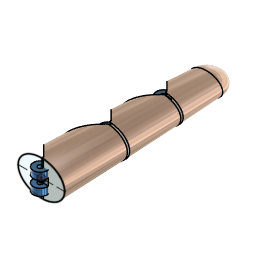
index finger assembly v3 (Autodesk Fusion 360 design; units mm, degrees)
Autodesk Fusion 360 part; units mm, degrees
sketch "base" plane through (0, 0, 0) normal (0, 1, 0) x (1, 0, 0) in component "index and ring finger part 2 v4"
  ellipse E0 centre (0, 0) end of major axis (9, 0) minor radius 6.5
  line L0 (-9, 0) -> (9, 0) construction
  line L1 (0, -6.5) -> (0, 6.5) construction
  dimension "d1" = 18
  dimension "d2" = 13
  constraint coincident E0 L0.start
  constraint coincident E0 L0.end
  constraint coincident E0 L1.start
  constraint coincident E0 L1.end
  constraint coincident E0.centre origin
  constraint horizontal L0
  measures "d1" distance of E0
ref_plane "WorkPlane1" through (0, 23, 0) normal (0, 1, 0) x (1, 0, 0) in component "index and ring finger part 2 v4"
sketch "top" plane through (0, 23, 0) normal (0, 1, 0) x (1, 0, 0) in component "index and ring finger part 2 v4"
  ellipse E0 centre (0, 0) end of major axis (8, 0) minor radius 5.5
  line L0 (-8, 0) -> (8, 0) construction
  line L1 (0, -5.5) -> (0, 5.5) construction
  dimension "d4" = 16
  dimension "d5" = 11
  constraint coincident E0 L0.start
  constraint coincident E0 L0.end
  constraint coincident E0 L1.start
  constraint coincident E0 L1.end
  constraint coincident E0.centre origin
  constraint horizontal L0
  measures "d4" distance of E0
loft "Loft1" add profiles "top", "base" section 1 section 2 makes body 1 in component "index and ring finger part 2 v4"
sketch "cut" plane through (0, 0, 0) normal (0, 0, 1) x (1, 0, 0) in component "index and ring finger part 2 v4"
  line L0 (0, 23) -> (0, 23.5)
  line L1 (0, 0) -> (0, 1)
  line L2 (0, 1) -> (-14.1421, 15.1421)
  line L3 (0, 1) -> (20, 1) construction
  line L4 (-14.1421, 15.1421) -> (-14.1421, 0)
  line L5 (-14.1421, 0) -> (0, 0)
  line L6 (0, 0) -> (0, -0.5)
  line L7 (0, 23) -> (0, 22)
  line L8 (0, 22) -> (-14.1421, 7.8579)
  line L9 (0, 22) -> (20, 22) construction
  line L10 (0, 23) -> (-11.4565, 23)
  line L11 (-11.4565, 23) -> (-14.1421, 7.8579)
  dimension "d6" = 0.5
  dimension "d7" = 1
  dimension "d8" = 135
  dimension "d9" = 20
  dimension "d10" = 0.5
  dimension "d11" = 1
  dimension "d12" = 135
  dimension "d13" = 20
  constraint vertical L0
  constraint coincident L1.start L5.end
  constraint vertical L1
  constraint horizontal L3
  constraint parallel L1 L4
  constraint perpendicular L1 L5
  constraint perpendicular L5 L6
  constraint parallel L0 L7
  constraint horizontal L9
  constraint perpendicular L7 L10
  measures "d6" distance of L0.start L0.end
  measures "d7" distance of L1.start L1.end
  measures "d8" angle of L2 L3
  measures "d9" distance of L1.end L2.end
  measures "d10" distance of L1.start L6.end
  measures "d11" distance of L0.start L7.end
  measures "d12" angle of L8 L9
  measures "d13" distance of L7.end L8.end
extrude "Extrude1" cut sketch "cut" along normal mid plane 40 contours L1 L2 L4 L5 L8 | L2 L7 L8 L10 L11 bodies 1 in component "index and ring finger part 2 v4"
sketch "wheel" plane through (0, 0, 0) normal (0, 0, 1) x (1, 0, 0) in component "index and ring finger part 2 v4"
  line L0 (0, 0) -> (0, -0.5)
  circle A0 centre (0, -0.5) radius 3
  circle A1 centre (0.0423, 23.5794) radius 3
  dimension "d16" = 0.5
  dimension "d17" = 6
  dimension "d18" = 6
  constraint coincident L0.start origin
  constraint vertical L0
  constraint coincident L0.end A0.centre
  measures "d16" distance of L0.start L0.end
  measures "d17" diameter of A0
  measures "d18" diameter of A1
extrude "Extrude2" add sketch "wheel" along normal mid plane 3 separate body contours A1 makes body 2 in component "index and ring finger part 2 v4"
extrude "Extrude3" cut sketch "wheel" along normal mid plane 3 contours A0 bodies 1 in component "index and ring finger part 2 v4"
sketch "lower wheel offset" plane through (0, 0, -1.5) normal (0, 0, 1) x (-1, 0, 0) in component "index and ring finger part 2 v4"
  line L0 (0, 0) -> (-2.958, 0)
  arc A0 (-2.958, 0) -> (1.2343, -2.2343) centre (0, 0.5) ccw
  line L1 (1.2343, -2.2343) -> (0, -1)
  line L2 (0, -1) -> (0, 0)
  circle A1 centre (0, 0.5) radius 3
  dimension "d23" = 6
  constraint concentric A0 A1
  measures "d23" diameter of A1
extrude "Extrude4" add sketch "lower wheel offset" against normal blind 3 separate body makes body 3 in component "index and ring finger part 2 v4"
sketch "lower wheel offset2" plane through (0, 0, 1.5) normal (0, 0, -1) x (1, 0, 0) in component "index and ring finger part 2 v4"
  line L0 (2.958, 0) -> (0, 0)
  line L1 (0, 0) -> (0, -1)
  line L2 (0, -1) -> (-1.2343, -2.2343)
  arc A0 (-1.2343, -2.2343) -> (2.958, 0) centre (0, 0.5) ccw
  circle A1 centre (0, 0.5) radius 3
  dimension "d26" = 6
  constraint concentric A0 A1
  measures "d26" diameter of A1
extrude "Extrude5" add sketch "lower wheel offset2" against normal blind 3 separate body makes body 4 in component "index and ring finger part 2 v4"
sketch "rod cut" plane through (0, 0, 0) normal (0, 0, 1) x (1, 0, 0) in component "index and ring finger part 2 v4"
  circle A0 centre (0, -0.5) radius 1
  circle A1 centre (0, 23.5) radius 1
  dimension "d29" = 2
  dimension "d30" = 2
  measures "d29" diameter of A0
  measures "d30" diameter of A1
extrude "Extrude6" cut sketch "rod cut" along normal mid plane 40 bodies 1 2 3 4 in component "index and ring finger part 2 v4"
sketch "cut1" plane through (0, 0, 0) normal (0, 0, 1) x (1, 0, 0) in component "index and ring finger part 2 v4"
  line L0 (-7.9545, 27.9627) -> (-8.9545, -0.0373)
  line L1 (-8.2576, 19.4763) -> (-8.7573, 19.4941)
  line L2 (-8.7573, 19.4941) -> (-9.1833, 7.5654)
  line L3 (-9.1833, 7.5654) -> (-6.6849, 7.4762)
  line L4 (-6.6849, 7.4762) -> (-6.1718, 21.8428)
  line L5 (-6.1718, 21.8428) -> (-9.5, 19.5225)
  dimension "d34" = 0.5
  dimension "d35" = 2.5
  constraint coincident L0 L1.start
  constraint perpendicular L0 L1
  constraint perpendicular L1 L2
  constraint perpendicular L0 L3
  constraint perpendicular L3 L4
  measures "d34" distance of L1.start L1.end
  measures "d35" distance of L2.end L3.end
extrude "Extrude7" cut sketch "cut1" along normal mid plane 2 bodies 1 in component "index and ring finger part 2 v4"
sketch "cut 2" plane through (0, 0, 0) normal (0, 0, 1) x (1, 0, 0) in component "index and ring finger part 2 v4"
  line L0 (-7.9187, 24.4013) -> (-8.9187, -3.5987)
  line L1 (-8.0516, 20.6796) -> (-7.552, 20.6618)
  line L2 (-7.552, 20.6618) -> (-7.9333, 9.9832)
  line L3 (-7.9333, 9.9832) -> (-6.934, 9.9475)
  line L4 (-6.934, 9.9475) -> (-6.6023, 19.2349)
  line L5 (-6.6023, 19.2349) -> (-7.552, 20.6618)
  dimension "d38" = 0.5
  dimension "d39" = 1
  constraint coincident L0 L1.start
  constraint perpendicular L0 L1
  constraint perpendicular L1 L2
  constraint perpendicular L2 L3
  constraint perpendicular L3 L4
  measures "d38" distance of L1.start L1.end
  measures "d39" distance of L2.end L3.end
extrude "Extrude8" cut sketch "cut 2" along normal mid plane 4 bodies 1 in component "index and ring finger part 2 v4"
copy_body "Body->Comp1" bodies 1 removing the originals makes body 5 in component "index part 1"
copy_body "Body->Comp2" bodies 2 removing the originals makes body 6 in component "uppr wheel"
copy_body "Body->Comp3" bodies 3 removing the originals makes body 7 in component "lower wheel 1"
copy_body "Body->Comp4" bodies 4 removing the originals makes body 8 in component "lower wheel 2"
sketch "Sketch11" plane through (0, 0, 0) normal (0, 1, 0) x (1, 0, 0) in component "index and ring finger part 2 v4"
extrude "Extrude1'" cut 1 faces at (0.7378, 25.769, 1.5) along direction (0, 0, 1) blind 3 on bodies 6 bodies 5 in component "index part 1"
extrude "Extrude2'" cut 1 faces at (0.7378, 25.769, -1.5) along direction (0, 0, -1) blind 3 on bodies 6 bodies 5 in component "index part 1"
combine "Combine1" operation add target body 5 tool bodies 8 7 6 in component "index part 1"
sketch "base (2)" plane through (0, 0, 0) normal (0, 1, 0) x (1, 0, 0) in component "index and ring finger part 3 v2"
  ellipse E0 centre (0, 0) end of major axis (8, 0) minor radius 5.5
  line L0 (-8, 0) -> (8, 0) construction
  line L1 (0, -5.5) -> (0, 5.5) construction
  dimension "d1_1" = 16
  dimension "d2_1" = 11
  constraint coincident E0 L0.start
  constraint coincident E0 L0.end
  constraint coincident E0 L1.start
  constraint coincident E0 L1.end
  constraint coincident E0.centre origin
  constraint horizontal L0
  measures "d1_1" distance of E0
ref_plane "WorkPlane1" through (0, 18, 0) normal (0, 1, 0) x (1, 0, 0) in component "index and ring finger part 3 v2"
sketch "top (2)" plane through (0, 18, 0) normal (0, 1, 0) x (1, 0, 0) in component "index and ring finger part 3 v2"
  ellipse E0 centre (0, 0) end of major axis (7, 0) minor radius 4.5
  line L0 (-7, 0) -> (7, 0) construction
  line L1 (0, -4.5) -> (0, 4.5) construction
  dimension "d4_1" = 14
  dimension "d5_1" = 9
  constraint coincident E0 L0.start
  constraint coincident E0 L0.end
  constraint coincident E0 L1.start
  constraint coincident E0 L1.end
  constraint coincident E0.centre origin
  constraint horizontal L0
  measures "d4_1" distance of E0
loft "Loft1'" add profiles "top (2)", "base (2)" section 1 section 2 separate body makes body 9 in component "index and ring finger part 3 v2"
sketch "cut (2)" plane through (0, 0, 0) normal (0, 0, 1) x (1, 0, 0) in component "index and ring finger part 3 v2"
  line L0 (0, 28) -> (0, 28.5)
  line L1 (0, 0) -> (0, 1)
  line L2 (0, 1) -> (-14.1421, 15.1421)
  line L3 (0, 1) -> (20, 1) construction
  line L4 (-14.1421, 15.1421) -> (-14.1421, 0)
  line L5 (-14.1421, 0) -> (0, 0)
  line L6 (0, 0) -> (0, -0.5)
  line L7 (0, 28) -> (0, 27)
  line L8 (0, 27) -> (20, 27) construction
  line L9 (0, 28) -> (-11.4565, 28)
  line L10 (-11.4565, 28) -> (-14.1421, 12.8579)
  dimension "d6_1" = 0.5
  dimension "d7_1" = 1
  dimension "d8_1" = 135
  dimension "d9_1" = 20
  dimension "d10_1" = 0.5
  dimension "d11_1" = 1
  dimension "d13_1" = 20
  constraint vertical L0
  constraint coincident L1.start L5.end
  constraint vertical L1
  constraint horizontal L3
  constraint parallel L1 L4
  constraint perpendicular L1 L5
  constraint perpendicular L5 L6
  constraint parallel L0 L7
  constraint horizontal L8
  constraint perpendicular L7 L9
  measures "d6_1" distance of L0.start L0.end
  measures "d7_1" distance of L1.start L1.end
  measures "d8_1" angle of L2 L3
  measures "d9_1" distance of L1.end L2.end
  measures "d10_1" distance of L1.start L6.end
  measures "d11_1" distance of L0.start L7.end
  measures "d13_1" distance of L7.end L10.end
extrude "Extrude1''" cut sketch "cut (2)" along normal mid plane 40 contours L1 L2 L4 L5 L10 bodies 9 in component "index and ring finger part 3 v2"
sketch "wheel (2)" plane through (0, 0, 0) normal (0, 0, 1) x (1, 0, 0) in component "index and ring finger part 3 v2"
  line L0 (0, 0) -> (0, -0.5)
  circle A0 centre (0, -0.5) radius 3
  dimension "d16_1" = 0.5
  dimension "d17_1" = 6
  constraint coincident L0.start origin
  constraint vertical L0
  constraint coincident L0.end A0.centre
  measures "d16_1" distance of L0.start L0.end
  measures "d17_1" diameter of A0
extrude "Extrude3'" cut sketch "wheel (2)" along normal mid plane 3 bodies 9 in component "index and ring finger part 3 v2"
sketch "lower wheel offset (2)" plane through (0, 0, -1.5) normal (0, 0, 1) x (-1, 0, 0) in component "index and ring finger part 3 v2"
  line L0 (0, 0) -> (-2.958, 0)
  arc A0 (-2.958, 0) -> (1.2343, -2.2343) centre (0, 0.5) ccw
  line L1 (0, -1) -> (0, 0)
  circle A1 centre (0, 0.5) radius 3
  line L2 (1.2343, -2.2343) -> (0, -1)
  dimension "d23_1" = 6
  constraint concentric A0 A1
  measures "d23_1" diameter of A1
extrude "Extrude4'" add sketch "lower wheel offset (2)" against normal blind 3 separate body makes body 10 in component "index and ring finger part 3 v2"
sketch "lower wheel offset2 (2)" plane through (0, 0, 1.5) normal (0, 0, -1) x (1, 0, 0) in component "index and ring finger part 3 v2"
  line L0 (2.958, 0) -> (0, 0)
  line L1 (0, 0) -> (0, -1)
  arc A0 (-1.2343, -2.2343) -> (2.958, 0) centre (0, 0.5) ccw
  circle A1 centre (0, 0.5) radius 3
  line L2 (0, -1) -> (-1.2343, -2.2343)
  dimension "d26_1" = 6
  constraint concentric A0 A1
  measures "d26_1" diameter of A1
extrude "Extrude5'" add sketch "lower wheel offset2 (2)" against normal blind 3 separate body makes body 11 in component "index and ring finger part 3 v2"
sketch "rod cut (2)" plane through (0, 0, 0) normal (0, 0, 1) x (1, 0, 0) in component "index and ring finger part 3 v2"
  circle A0 centre (0, -0.5) radius 1
  dimension "d29_1" = 2
  measures "d29_1" diameter of A0
copy_body "Body->Comp1'" bodies 9 removing the originals makes body 12 in component "index part 1 (1)"
copy_body "Body->Comp3'" bodies 10 removing the originals makes body 13 in component "lower wheel 1 (1)"
copy_body "Body->Comp4'" bodies 11 removing the originals makes body 14 in component "lower wheel 2 (1)"
sketch "Sketch12" plane through (0, 18, 0) normal (0, 1, 0) x (-1, 0, 0) in component "index and ring finger part 3 v2"
  ellipse E0 centre (0, 0) end of major axis (-7, 0) minor radius 4.5
  line L0 (0, -4.5) -> (0, 4.5)
  ellipse E1 centre (0, 0) end of major axis (-7, 0) minor radius 4.5 (0, 4.5) -> (0, -4.5) ccw
  dimension "d46" = 14
  dimension "d47" = 9
  constraint coincident E0.centre E1.centre
  measures "d46" distance of E1
revolve "Revolve1" add sketch "Sketch12" angle 180 about axis through (0, 18, -4.5) along (0, 0, 1) contours E0 L0 E1 bodies 12 in component "index part 1 (1)"
extrude "Extrude3''" cut sketch "rod cut (2)" along normal mid plane 40 bodies 12 in component "index part 1 (1)"
extrude "Extrude1'''" cut sketch "rod cut (2)" along normal mid plane 40 bodies 13 in component "lower wheel 1 (1)"
extrude "Extrude1''''" cut sketch "rod cut (2)" along normal mid plane 40 bodies 14 in component "lower wheel 2 (1)"
combine "Combine1'" operation add target body 12 tool bodies 13 14 in component "index part 1 (1)"
sketch "base (3)" plane through (0, 0, 0) normal (0, 1, 0) x (1, 0, 0) in component "index and ring finger part 1(incorrect) v6"
  ellipse E0 centre (0, 0) end of major axis (10, 0) minor radius 7.5
  line L0 (-10, 0) -> (10, 0) construction
  line L1 (0, -7.5) -> (0, 7.5) construction
  dimension "d1_2" = 20
  dimension "d2_2" = 15
  constraint coincident E0 L0.start
  constraint coincident E0 L0.end
  constraint coincident E0 L1.start
  constraint coincident E0 L1.end
  constraint coincident E0.centre origin
  constraint horizontal L0
  measures "d1_2" distance of E0
ref_plane "WorkPlane1" through (0, 28, 0) normal (0, 1, 0) x (1, 0, 0) in component "index and ring finger part 1(incorrect) v6"
sketch "top (3)" plane through (0, 28, 0) normal (0, 1, 0) x (1, 0, 0) in component "index and ring finger part 1(incorrect) v6"
  ellipse E0 centre (0, 0) end of major axis (9, 0) minor radius 6.5
  line L0 (-9, 0) -> (9, 0) construction
  line L1 (0, -6.5) -> (0, 6.5) construction
  dimension "d4_2" = 18
  dimension "d5_2" = 13
  constraint coincident E0 L0.start
  constraint coincident E0 L0.end
  constraint coincident E0 L1.start
  constraint coincident E0 L1.end
  constraint coincident E0.centre origin
  constraint horizontal L0
  measures "d4_2" distance of E0
loft "Loft1''" add profiles "top (3)", "base (3)" section 1 section 2 separate body makes body 15 in component "index and ring finger part 1(incorrect) v6"
sketch "cut (3)" plane through (0, 0, 0) normal (0, 0, 1) x (1, 0, 0) in component "index and ring finger part 1(incorrect) v6"
  line L0 (0, 28) -> (0, 28.5)
  line L1 (0, 0) -> (0, 1)
  line L2 (0, 1) -> (-14.1421, 15.1421)
  line L3 (0, 1) -> (20, 1) construction
  line L4 (-14.1421, 15.1421) -> (-14.1421, 0)
  line L5 (-14.1421, 0) -> (0, 0)
  line L6 (0, 0) -> (0, -0.5)
  line L7 (0, 28) -> (0, 27)
  line L8 (0, 27) -> (-14.1421, 12.8579)
  line L9 (0, 27) -> (20, 27) construction
  line L10 (0, 28) -> (-11.4565, 28)
  line L11 (-11.4565, 28) -> (-14.1421, 12.8579)
  dimension "d6_2" = 0.5
  dimension "d7_2" = 1
  dimension "d8_2" = 135
  dimension "d9_2" = 20
  dimension "d10_2" = 0.5
  dimension "d11_2" = 1
  dimension "d12_1" = 135
  dimension "d13_2" = 20
  constraint vertical L0
  constraint coincident L1.start L5.end
  constraint vertical L1
  constraint horizontal L3
  constraint parallel L1 L4
  constraint perpendicular L1 L5
  constraint perpendicular L5 L6
  constraint parallel L0 L7
  constraint horizontal L9
  constraint perpendicular L7 L10
  measures "d6_2" distance of L0.start L0.end
  measures "d7_2" distance of L1.start L1.end
  measures "d8_2" angle of L2 L3
  measures "d9_2" distance of L1.end L2.end
  measures "d10_2" distance of L1.start L6.end
  measures "d11_2" distance of L0.start L7.end
  measures "d12_1" angle of L8 L9
  measures "d13_2" distance of L7.end L8.end
extrude "Extrude1'''''" cut sketch "cut (3)" along normal mid plane 40 contours L1 L2 L4 L5 L8 | L2 L7 L8 L10 L11 bodies 15 in component "index and ring finger part 1(incorrect) v6"
sketch "wheel (3)" plane through (0, 0, 0) normal (0, 0, 1) x (1, 0, 0) in component "index and ring finger part 1(incorrect) v6"
  line L0 (0, 0) -> (0, -0.5)
  circle A0 centre (0, -0.5) radius 3
  circle A1 centre (0.0423, 28.5794) radius 3
  dimension "d16_2" = 0.5
  dimension "d17_2" = 6
  dimension "d18_1" = 6
  constraint coincident L0.start origin
  constraint vertical L0
  constraint coincident L0.end A0.centre
  measures "d16_2" distance of L0.start L0.end
  measures "d17_2" diameter of A0
  measures "d18_1" diameter of A1
extrude "Extrude2''" add sketch "wheel (3)" along normal mid plane 3 separate body contours A1 makes body 16 in component "index and ring finger part 1(incorrect) v6"
extrude "Extrude3'''" cut sketch "wheel (3)" along normal mid plane 3 contours A0 bodies 15 in component "index and ring finger part 1(incorrect) v6"
sketch "lower wheel offset (3)" plane through (0, 0, -1.5) normal (0, 0, 1) x (-1, 0, 0) in component "index and ring finger part 1(incorrect) v6"
  line L0 (0, 0) -> (-2.958, 0)
  arc A0 (-2.958, 0) -> (1.2343, -2.2343) centre (0, 0.5) ccw
  line L1 (1.2343, -2.2343) -> (0, -1)
  line L2 (0, -1) -> (0, 0)
  circle A1 centre (0, 0.5) radius 3
  dimension "d23_2" = 6
  constraint concentric A0 A1
  measures "d23_2" diameter of A1
extrude "Extrude4''" add sketch "lower wheel offset (3)" against normal blind 3 separate body makes body 17 in component "index and ring finger part 1(incorrect) v6"
sketch "lower wheel offset2 (3)" plane through (0, 0, 1.5) normal (0, 0, -1) x (1, 0, 0) in component "index and ring finger part 1(incorrect) v6"
  line L0 (2.958, 0) -> (0, 0)
  line L1 (0, 0) -> (0, -1)
  line L2 (0, -1) -> (-1.2343, -2.2343)
  arc A0 (-1.2343, -2.2343) -> (2.958, 0) centre (0, 0.5) ccw
  circle A1 centre (0, 0.5) radius 3
  dimension "d26_2" = 6
  constraint concentric A0 A1
  measures "d26_2" diameter of A1
extrude "Extrude5''" add sketch "lower wheel offset2 (3)" against normal blind 3 separate body makes body 18 in component "index and ring finger part 1(incorrect) v6"
sketch "rod cut (3)" plane through (0, 0, 0) normal (0, 0, 1) x (1, 0, 0) in component "index and ring finger part 1(incorrect) v6"
  circle A0 centre (0, -0.5) radius 1
  circle A1 centre (0, 28.5) radius 1
  dimension "d29_2" = 2
  dimension "d30_1" = 2
  measures "d29_2" diameter of A0
  measures "d30_1" diameter of A1
extrude "Extrude6'" cut sketch "rod cut (3)" along normal mid plane 40 bodies 15 16 17 18 in component "index and ring finger part 1(incorrect) v6"
sketch "cut1 (2)" plane through (0, 0, 0) normal (0, 0, 1) x (1, 0, 0) in component "index and ring finger part 1(incorrect) v6"
  line L0 (-9, 28) -> (-10, 0)
  line L1 (-9.3031, 19.5136) -> (-9.8028, 19.5314)
  line L2 (-9.8028, 19.5314) -> (-10.196, 8.5218)
  line L3 (-10.196, 8.5218) -> (-7.6976, 8.4326)
  line L4 (-7.6976, 8.4326) -> (-7.2421, 21.1848)
  line L5 (-7.2421, 21.1848) -> (-9.5, 19.5225)
  dimension "d34_1" = 0.5
  dimension "d35_1" = 2.5
  constraint coincident L0 L1.start
  constraint perpendicular L0 L1
  constraint perpendicular L1 L2
  constraint perpendicular L0 L3
  constraint perpendicular L3 L4
  measures "d34_1" distance of L1.start L1.end
  measures "d35_1" distance of L2.end L3.end
extrude "Extrude7'" cut sketch "cut1 (2)" along normal mid plane 2 contours L0 L3 L4 L5 | L0 L1 L2 L3 bodies 15 in component "index and ring finger part 1(incorrect) v6"
sketch "cut 2 (2)" plane through (0, 0, 0) normal (0, 0, 1) x (1, 0, 0) in component "index and ring finger part 1(incorrect) v6"
  line L0 (-9, 28) -> (-10, 0)
  line L1 (-9.2187, 21.8761) -> (-8.719, 21.8582)
  line L2 (-8.719, 21.8582) -> (-9.1005, 11.1785)
  line L3 (-9.1005, 11.1785) -> (-8.1011, 11.1428)
  line L4 (-8.1011, 11.1428) -> (-7.7659, 20.5294)
  line L5 (-7.7659, 20.5294) -> (-8.719, 21.8582)
  dimension "d38_1" = 0.5
  dimension "d39_1" = 1
  constraint coincident L0 L1.start
  constraint perpendicular L0 L1
  constraint perpendicular L1 L2
  constraint perpendicular L2 L3
  constraint perpendicular L3 L4
  measures "d38_1" distance of L1.start L1.end
  measures "d39_1" distance of L2.end L3.end
extrude "Extrude8'" cut sketch "cut 2 (2)" along normal mid plane 4 bodies 15 in component "index and ring finger part 1(incorrect) v6"
copy_body "Body->Comp1''" bodies 15 removing the originals makes body 19 in component "index part 1 (2)"
copy_body "Body->Comp2'" bodies 16 removing the originals makes body 20 in component "uppr wheel (1)"
copy_body "Body->Comp3''" bodies 17 removing the originals makes body 21 in component "lower wheel 1 (2)"
copy_body "Body->Comp4''" bodies 18 removing the originals makes body 22 in component "lower wheel 2 (2)"
sketch "Sketch11 (2)" plane through (0, 0, 0) normal (0, 1, 0) x (1, 0, 0) in component "index and ring finger part 1(incorrect) v6"
component "index and ring finger part 2 v4" placed x (1, 0, 0) y (0, 1, 0) z (0, 0, 1) at (0, 0, 0)
component "index and ring finger part 3 v2" placed x (1, 0, 0) y (0, 1, 0) z (0, 0, 1) at (0, 0, 0)
component "index and ring finger part 1(incorrect) v6" placed x (1, 0, 0) y (0, 1, 0) z (0, 0, 1) at (0, 0, 0)
component "index part 1" placed x (1, 0, 0) y (0, 1, 0) z (0, 0, 1) at (0, 29, 0) in component "index and ring finger part 2 v4"
component "uppr wheel" placed x (1, 0, 0) y (0, 1, 0) z (0, 0, 1) at (0, 0, 0) in component "index and ring finger part 2 v4"
component "lower wheel 1" placed x (1, 0, 0) y (0, 1, 0) z (0, 0, 1) at (0, 0, 0) in component "index and ring finger part 2 v4"
component "lower wheel 2" placed x (1, 0, 0) y (0, 1, 0) z (0, 0, 1) at (0, 0, 0) in component "index and ring finger part 2 v4"
component "index part 1 (1)" placed x (1, 0, 0) y (0, 1, 0) z (0, 0, 1) at (0, 53, 0) in component "index and ring finger part 3 v2"
component "lower wheel 1 (1)" placed x (1, 0, 0) y (0, 1, 0) z (0, 0, 1) at (0, 0, 0) in component "index and ring finger part 3 v2"
component "lower wheel 2 (1)" placed x (1, 0, 0) y (0, 1, 0) z (0, 0, 1) at (0, 0, 0) in component "index and ring finger part 3 v2"
component "index part 1 (2)" placed x (1, 0, 0) y (0, 1, 0) z (0, 0, 1) at (0, 0, 0) in component "index and ring finger part 1(incorrect) v6"
component "uppr wheel (1)" placed x (1, 0, 0) y (0, 1, 0) z (0, 0, 1) at (0, 0, 0) in component "index and ring finger part 1(incorrect) v6"
component "lower wheel 1 (2)" placed x (1, 0, 0) y (0, 1, 0) z (0, 0, 1) at (0, 0, 0) in component "index and ring finger part 1(incorrect) v6"
component "lower wheel 2 (2)" placed x (1, 0, 0) y (0, 1, 0) z (0, 0, 1) at (0, 0, 0) in component "index and ring finger part 1(incorrect) v6"
named bodies: "index part 1", "uppr wheel", "lower wheel 1", "lower wheel 2"
